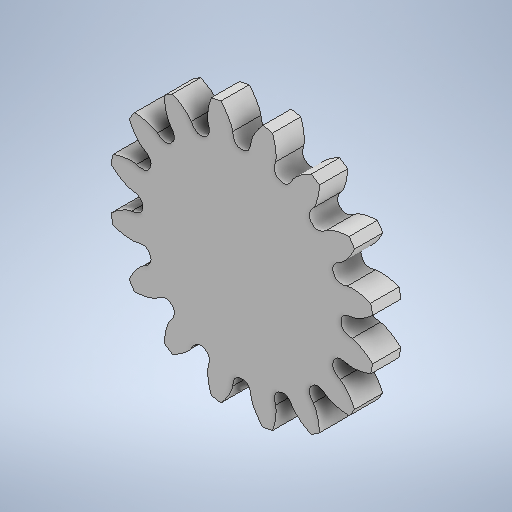
# Autodesk Inventor part: small gear
Saved by Autodesk Inventor 2025 (Build 290162010, 162A)
## iProperties
Created: 2025-08-27
Part Number: small gear
Material: Generic
Document SubType Name: Modeling
Designer: pokla
Density: 1 g/cm^3
Appearance: Default
Author: pokla
Autodesk Inventor part; units mm, degrees
ref_plane "YZ Plane" through (0, 0, 0) normal (1, 0, 0) x (0, 1, 0)
ref_plane "XZ Plane" through (0, 0, 0) normal (0, 1, 0) x (-1, 0, 0)
ref_plane "XY Plane" through (0, 0, 0) normal (0, 0, 1) x (1, 0, 0)
sketch "Sketch1" plane through (0, 0, 0) normal (0, 0, 1) x (1, 0, 0)
  spline S0 degree 3 poles (-17.8508, 111.0747) (-17.285, 110.4428) (-16.1535, 109.1789) (-14.5639, 107.1908) (-13.0641, 105.1347) (-11.6747, 103.0019) (-10.4104, 100.7926) (-9.4822, 98.8844) (-8.8332, 97.3167) (-8.4066, 96.1183) (-8.0336, 94.9) (-7.8885, 94.0639) (-7.816, 93.646) knots 0 0 0 0 0.254419 0.508838 0.763254 1.017664 1.272064 1.526448 1.653658 1.780865 1.908061 2.035185 2.035185 2.035185 2.035185
  spline S1 degree 3 poles (-7.816, 93.646) (-7.7696, 93.0759) (-7.7, 92.2205) (-7.5111, 91.0915) (-7.3096, 90.2571) (-7.0647, 89.4342) (-6.7496, 88.6354) (-6.3767, 87.8619) (-5.9264, 87.1299) (-5.3982, 86.4517) (-4.7906, 85.8433) (-4.109, 85.319) (-3.362, 84.8917) (-2.5584, 84.5833) (-1.7166, 84.3988) (-0.8573, 84.3642) (0, 84.3804) (0.8573, 84.3642) (1.7166, 84.3988) (2.5584, 84.5833) (3.362, 84.8917) (4.109, 85.319) (4.7906, 85.8433) (5.3982, 86.4517) (5.9264, 87.1299) (6.3767, 87.8619) (6.7496, 88.6354) (7.0647, 89.4342) (7.3096, 90.2571) (7.5111, 91.0915) (7.7, 92.2205) (7.7696, 93.0759) (7.816, 93.646) knots 0 0 0 0 0.17153 0.25732 0.343104 0.428894 0.514663 0.600431 0.686214 0.771984 0.857728 0.943463 1.029224 1.114985 1.200743 1.286467 1.372253 1.45804 1.543764 1.629522 1.715283 1.801044 1.886779 1.972523 2.058293 2.144076 2.229844 2.315613 2.401403 2.487187 2.572976 2.744507 2.744507 2.744507 2.744507
  spline S2 degree 3 poles (7.816, 93.646) (7.8885, 94.0639) (8.0336, 94.9) (8.4066, 96.1183) (8.8332, 97.3167) (9.4822, 98.8844) (10.4104, 100.7926) (11.6747, 103.0019) (13.0641, 105.1347) (14.5639, 107.1908) (16.1535, 109.1789) (17.285, 110.4428) (17.8508, 111.0747) knots 0 0 0 0 0.127124 0.25432 0.381527 0.508737 0.763121 1.017521 1.271931 1.526346 1.780766 2.035185 2.035185 2.035185 2.035185
  circle A0 centre (0, 0) radius 84.375 construction
  circle A1 centre (0, 0) radius 93.9693 construction
  circle A2 centre (0, 0) radius 100 construction
  circle A3 centre (0, 0) radius 112.5
  point P0 (-16.1714, 109.1636)
  point P1 (-14.5789, 107.1795)
  point P2 (-13.0825, 105.1219)
  point P3 (-11.6955, 102.9891)
  point P4 (-10.4354, 100.7791)
  point P5 (-9.3278, 98.4891)
  point P6 (-8.8432, 97.3129)
  point P7 (-8.4155, 96.1149)
  point P8 (-8.0594, 94.8938)
  point P9 (-7.6448, 91.9393)
  point P10 (-7.5011, 91.0935)
  point P11 (-7.3024, 90.259)
  point P12 (-7.053, 89.4382)
  point P13 (-6.74, 88.6396)
  point P14 (-6.3638, 87.8689)
  point P15 (-5.9134, 87.1388)
  point P16 (-5.3849, 86.4633)
  point P17 (-4.7783, 85.8573)
  point P18 (-4.0982, 85.3352)
  point P19 (-3.3526, 84.9115)
  point P20 (-2.552, 84.604)
  point P21 (-1.7136, 84.4237)
  point P22 (-0.8579, 84.3726)
  point P23 (0, 84.375)
  point P24 (0.8579, 84.3726)
  point P25 (1.7136, 84.4237)
  point P26 (2.552, 84.604)
  point P27 (3.3526, 84.9115)
  point P28 (4.0982, 85.3352)
  point P29 (4.7783, 85.8573)
  point P30 (5.3849, 86.4633)
  point P31 (5.9134, 87.1388)
  point P32 (6.3638, 87.8689)
  point P33 (6.74, 88.6396)
  point P34 (7.053, 89.4382)
  point P35 (7.3024, 90.259)
  point P36 (7.5011, 91.0935)
  point P37 (7.6448, 91.9393)
  point P38 (8.0594, 94.8938)
  point P39 (8.4155, 96.1149)
  point P40 (8.8432, 97.3129)
  point P41 (9.3278, 98.4891)
  point P42 (10.4354, 100.7791)
  point P43 (11.6955, 102.9891)
  point P44 (13.0825, 105.1219)
  point P45 (14.5789, 107.1795)
  point P46 (16.1714, 109.1636)
  constraints: 4 centre point, 2 point on circle, 109 other
extrude "Extrusion1" add sketch "Sketch1" against normal blind 24
extrude "Extrusion2" cut sketch "Sketch1" against normal through all contours A3 S2 S1 S0 picked at (1.8307, 103.0835)
pattern_circular "Circular Pattern1" count 16 over 360 about axis through (0, 0, -10) along (0, 0, 1) of "Extrusion2"
equation "\"Module\" = 12.5"
equation "\"PressureAngle\" = 20deg"
equation "\"UnitProfileClearance\" = 0.25"
equation "\"UnitRoundRadius\" = 0.35"
equation "\"HeadDiameter\" = 225"
equation "\"RootDiameter\" = 168.75"
equation "\"BaseDiameter\" = 187.93852"
equation "\"HelixAngle\" = 0"
equation "\"UnitCorrection\" = 0"
equation "\"UnitAddendumModification\" = 0"
equation "\"CircularPitch\" = 39.269908"
equation "\"UnitBacklashShift\" = 0"
equation "\"TotalToolShift\" = 0"
equation "\"IsInternal\" = 0"
body "Solid1"
